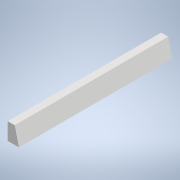
# Autodesk Inventor part: RearBumperFill
Saved by Autodesk Inventor 2020 (Build 240168000, 168)
## iProperties
Created: 2020-01-19
Part Number: RearBumperFill
Material: Generic
Document SubType Name: Modeling
Designer: srini
Density: 1 g/cm^3
Appearance: Default
Author: srini
Autodesk Inventor part; units mm, degrees
ref_plane "YZ Plane" through (0, 0, 0) normal (1, 0, 0) x (0, 1, 0)
ref_plane "XZ Plane" through (0, 0, 0) normal (0, 1, 0) x (-1, 0, 0)
sketch "Sketch1" plane through (0, 0, 0) normal (0, 0, 1) x (1, 0, 0)
  line L0 (-812.8, -3.937) -> (0, -3.937) projected
  line L1 (0, 73.787) -> (-812.8, 73.787) projected
  line L2 (-813.562, 73.533) -> (-813.562, -3.175) projected
  line L3 (-762.762, -3.937) -> (-762.762, -7.112) projected
  line L4 (-781.812, 77.47) -> (-781.812, 74.295) projected
  line L5 (-762.762, -3.937) -> (-813.562, -3.937)
  line L6 (-813.562, -3.937) -> (-813.562, 73.787)
  line L7 (-813.562, 73.787) -> (-781.6883, 73.787)
  line L8 (-781.6883, 73.787) -> (-762.762, -3.937)
  point P0 (0, 0)
  constraints: 8 end point, 3 collinear, 3 point on line, 2 perpendicular, 1 horizontal
ref_plane "Work Plane1" through (-812.8, 0, -698.5) normal (0, 0, -1) x (0, 1, 0)
extrude "Extrusion1" add sketch "Sketch1" against normal up to surface (698.5 mm away)
body "Solid1"
